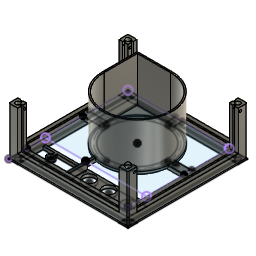
frame_top (Autodesk Fusion 360 design; units mm, degrees)
Autodesk Fusion 360 part; units mm, degrees
note: some values were not read from the file. Set by a fixed rule: which sketch regions a step uses.
sketch "Skizze1" plane through (0, 0, 0) normal (0, 0, 1) x (1, 0, 0)
  line L0 (0, 0) -> (160, 0)
  line L1 (160, 0) -> (160, 160)
  line L2 (160, 160) -> (0, 160)
  line L3 (0, 160) -> (0, 0)
  line L4 (0, 0) -> (12, 0)
  line L5 (12, 0) -> (12, 12)
  line L6 (12, 12) -> (0, 12)
  line L7 (0, 12) -> (0, 0)
  line L8 (160, 0) -> (148, 0)
  line L9 (148, 0) -> (148, 12)
  line L10 (148, 12) -> (160, 12)
  line L11 (160, 12) -> (160, 0)
  line L12 (160, 160) -> (148, 160)
  line L13 (148, 160) -> (148, 148)
  line L14 (148, 148) -> (160, 148)
  line L15 (160, 148) -> (160, 160)
  line L16 (0, 160) -> (12, 160)
  line L17 (12, 160) -> (12, 148)
  line L18 (12, 148) -> (0, 148)
  line L19 (0, 148) -> (0, 160)
  line L20 (12, 148) -> (148, 148)
  line L21 (148, 148) -> (148, 12)
  line L22 (148, 12) -> (12, 12)
  line L23 (12, 12) -> (12, 148)
  circle A0 centre (154, 154) radius 3
  circle A1 centre (6, 154) radius 3
  circle A2 centre (6, 6) radius 3
  circle A3 centre (154, 6) radius 3
  line L24 (4.9, 148) -> (7.1, 148)
  line L25 (7.1, 148) -> (7.1, 12)
  line L26 (7.1, 12) -> (4.9, 12)
  line L27 (4.9, 12) -> (4.9, 148)
  line L28 (152.9, 148) -> (155.1, 148)
  line L29 (155.1, 148) -> (155.1, 12)
  line L30 (155.1, 12) -> (152.9, 12)
  line L31 (152.9, 12) -> (152.9, 148)
  line L32 (12, 155.1) -> (148, 155.1)
  line L33 (148, 155.1) -> (148, 152.9)
  line L34 (148, 152.9) -> (12, 152.9)
  line L35 (12, 152.9) -> (12, 155.1)
  line L36 (12, 7.1) -> (148, 7.1)
  line L37 (148, 7.1) -> (148, 4.9)
  line L38 (148, 4.9) -> (12, 4.9)
  line L39 (12, 4.9) -> (12, 7.1)
  line L40 (148, 155.1) -> (150, 155.1)
  line L41 (150, 155.1) -> (150, 152.9)
  line L42 (150, 152.9) -> (148, 152.9)
  line L43 (148, 152.9) -> (148, 155.1)
  line L44 (152.9, 148) -> (155.1, 148)
  line L45 (155.1, 148) -> (155.1, 150)
  line L46 (155.1, 150) -> (152.9, 150)
  line L47 (152.9, 150) -> (152.9, 148)
  line L48 (12, 155.1) -> (10, 155.1)
  line L49 (10, 155.1) -> (10, 152.9)
  line L50 (10, 152.9) -> (12, 152.9)
  line L51 (12, 152.9) -> (12, 155.1)
  line L52 (4.9, 148) -> (7.1, 148)
  line L53 (7.1, 148) -> (7.1, 150)
  line L54 (7.1, 150) -> (4.9, 150)
  line L55 (4.9, 150) -> (4.9, 148)
  line L56 (12, 4.9) -> (10, 4.9)
  line L57 (10, 4.9) -> (10, 7.1)
  line L58 (10, 7.1) -> (12, 7.1)
  line L59 (12, 7.1) -> (12, 4.9)
  line L60 (4.9, 12) -> (7.1, 12)
  line L61 (7.1, 12) -> (7.1, 10)
  line L62 (7.1, 10) -> (4.9, 10)
  line L63 (4.9, 10) -> (4.9, 12)
  line L64 (148, 4.9) -> (150, 4.9)
  line L65 (150, 4.9) -> (150, 7.1)
  line L66 (150, 7.1) -> (148, 7.1)
  line L67 (148, 7.1) -> (148, 4.9)
  line L68 (152.9, 12) -> (155.1, 12)
  line L69 (155.1, 12) -> (155.1, 10)
  line L70 (155.1, 10) -> (152.9, 10)
  line L71 (152.9, 10) -> (152.9, 12)
  line L72 (148, 17) -> (66, 17)
  line L73 (66, 17) -> (66, 37)
  line L74 (66, 37) -> (148, 37)
  line L75 (148, 37) -> (148, 17)
  circle A4 centre (133, 27) radius 8.1
  circle A5 centre (107, 27) radius 8.1
  circle A6 centre (81, 27) radius 8.1
  line L76 (66, 37) -> (12, 37)
  line L77 (12, 37) -> (12, 34)
  line L78 (12, 34) -> (66, 34)
  line L79 (66, 34) -> (66, 37)
  line L80 (66, 17) -> (12, 17)
  line L81 (12, 17) -> (12, 20)
  line L82 (12, 20) -> (66, 20)
  line L83 (66, 20) -> (66, 17)
  circle A7 centre (29, 27) radius 3.6
  circle A8 centre (29, 27) radius 5
  line L84 (27.5, 34) -> (30.5, 34)
  line L85 (30.5, 34) -> (30.5, 12)
  line L86 (30.5, 12) -> (27.5, 12)
  line L87 (27.5, 12) -> (27.5, 34)
  dimension "d1" = 160
  dimension "d2" = 160
  dimension "d3" = 12
  dimension "d4" = 12
  dimension "d5" = 12
  dimension "d6" = 12
  dimension "d7" = 12
  dimension "d8" = 12
  dimension "d9" = 12
  dimension "d10" = 12
  dimension "d11" = 136
  dimension "d12" = 136
  dimension "d13" = 6
  dimension "d14" = 6
  dimension "d15" = 6
  dimension "d16" = 6
  dimension "d17" = 6
  dimension "d18" = 6
  dimension "d19" = 6
  dimension "d20" = 6
  dimension "d21" = 6
  dimension "d22" = 6
  dimension "d23" = 6
  dimension "d24" = 6
  dimension "d25" = 2.2
  dimension "d26" = 136
  dimension "d27" = 4.9
  dimension "d28" = 2.2
  dimension "d29" = 136
  dimension "d30" = 4.9
  dimension "d31" = 136
  dimension "d32" = 2.2
  dimension "d33" = 4.9
  dimension "d34" = 136
  dimension "d35" = 2.2
  dimension "d36" = 4.9
  dimension "d37" = 2
  dimension "d38" = 2.2
  dimension "d39" = 2.2
  dimension "d40" = 2
  dimension "d41" = 2
  dimension "d42" = 2.2
  dimension "d43" = 2.2
  dimension "d44" = 2
  dimension "d45" = 2
  dimension "d46" = 2.2
  dimension "d47" = 2.2
  dimension "d48" = 2
  dimension "d49" = 2
  dimension "d50" = 2.2
  dimension "d51" = 2.2
  dimension "d52" = 2
  dimension "d53" = 82
  dimension "d54" = 20
  dimension "d55" = 37
  dimension "d56" = 16.2
  dimension "d57" = 16.2
  dimension "d58" = 16.2
  dimension "d59" = 10
  dimension "d60" = 10
  dimension "d61" = 10
  dimension "d62" = 15
  dimension "d63" = 26
  dimension "d64" = 26
  dimension "d65" = 3
  dimension "d66" = 54
  dimension "d67" = 3
  dimension "d68" = 7.2
  dimension "d69" = 10
  dimension "d70" = 17
  dimension "d71" = 10
  dimension "d72" = 3
  dimension "d73" = 15.5
  constraint horizontal L0
  constraint vertical L1
  constraint horizontal L2
  constraint vertical L3
  constraint coincident L0.start L3.end
  constraint horizontal L4
  constraint vertical L5
  constraint horizontal L6
  constraint vertical L7
  constraint horizontal L8
  constraint vertical L9
  constraint horizontal L10
  constraint vertical L11
  constraint horizontal L12
  constraint vertical L13
  constraint horizontal L14
  constraint vertical L15
  constraint horizontal L16
  constraint vertical L17
  constraint horizontal L18
  constraint vertical L19
  constraint horizontal L20
  constraint vertical L21
  constraint horizontal L22
  constraint vertical L23
  constraint horizontal L24
  constraint vertical L25
  constraint horizontal L26
  constraint vertical L27
  constraint coincident L18 L24.start
  constraint horizontal L28
  constraint vertical L29
  constraint horizontal L30
  constraint vertical L31
  constraint coincident L14 L28.start
  constraint horizontal L32
  constraint vertical L33
  constraint horizontal L34
  constraint vertical L35
  constraint coincident L17 L32.start
  constraint horizontal L36
  constraint vertical L37
  constraint horizontal L38
  constraint vertical L39
  constraint coincident L5 L36.start
  constraint horizontal L40
  constraint vertical L41
  constraint horizontal L42
  constraint vertical L43
  constraint horizontal L44
  constraint vertical L45
  constraint horizontal L46
  constraint vertical L47
  constraint horizontal L48
  constraint vertical L49
  constraint horizontal L50
  constraint vertical L51
  constraint horizontal L52
  constraint vertical L53
  constraint horizontal L54
  constraint vertical L55
  constraint horizontal L56
  constraint vertical L57
  constraint horizontal L58
  constraint vertical L59
  constraint horizontal L60
  constraint vertical L61
  constraint horizontal L62
  constraint vertical L63
  constraint horizontal L64
  constraint vertical L65
  constraint horizontal L66
  constraint vertical L67
  constraint horizontal L68
  constraint vertical L69
  constraint horizontal L70
  constraint vertical L71
  constraint horizontal L72
  constraint vertical L73
  constraint horizontal L74
  constraint vertical L75
  constraint coincident L21 L72.start
  constraint horizontal L76
  constraint vertical L77
  constraint horizontal L78
  constraint vertical L79
  constraint horizontal L80
  constraint vertical L81
  constraint horizontal L82
  constraint vertical L83
  constraint concentric A7 A8
  constraint horizontal L84
  constraint vertical L85
  constraint horizontal L86
  constraint vertical L87
  constraint coincident L78 L84.start
  measures "d1" distance of L1 L3
  measures "d2" distance of L0 L2
  measures "d3" distance of L0.start L4.end
  measures "d4" distance of L0.start L6.end
  measures "d5" distance of L0.end L8.end
  measures "d6" distance of L0.end L10.end
  measures "d7" distance of L1.end L12.end
  measures "d8" distance of L1.end L14.end
  measures "d9" distance of L2.end L16.end
  measures "d10" distance of L2.end L18.end
  measures "d11" distance of L17.end L13.end
  measures "d12" distance of L17.end L5.end
  measures "d13" diameter of A0
  measures "d14" diameter of A1
  measures "d15" diameter of A2
  measures "d16" diameter of A3
  measures "d17" distance of L2 A0.centre
  measures "d18" distance of L15 A0.centre
  measures "d19" distance of L1 A3.centre
  measures "d20" distance of L8 A3.centre
  measures "d21" distance of L3 A2.centre
  measures "d22" distance of L4 A2.centre
  measures "d23" distance of L19 A1.centre
  measures "d24" distance of L2 A1.centre
  measures "d25" distance of L24.start L24.end
  measures "d26" distance of L24.start L26.end
  measures "d27" distance of L3 L27
  measures "d28" distance of L28.start L28.end
  measures "d29" distance of L28.start L30.end
  measures "d30" distance of L1 L29
  measures "d31" distance of L32.start L32.end
  measures "d32" distance of L32.start L34.end
  measures "d33" distance of L2 L32
  measures "d34" distance of L36.start L36.end
  measures "d35" distance of L36.start L38.end
  measures "d36" distance of L0 L38
  measures "d37" distance of L32.end L40.end
  measures "d38" distance of L32.end L33.end
  measures "d39" distance of L28.start L28.end
  measures "d40" distance of L28.start L46.end
  measures "d41" distance of L32.start L48.end
  measures "d42" distance of L32.start L34.end
  measures "d43" distance of L24.start L24.end
  measures "d44" distance of L24.start L54.end
  measures "d45" distance of L38.end L56.end
  measures "d46" distance of L38.end L36.start
  measures "d47" distance of L26.end L25.end
  measures "d48" distance of L26.end L62.end
  measures "d49" distance of L37.end L64.end
  measures "d50" distance of L37.end L36.end
  measures "d51" distance of L30.end L29.end
  measures "d52" distance of L30.end L70.end
  measures "d53" distance of L72.start L72.end
  measures "d54" distance of L72.start L74.end
  measures "d55" distance of L0 L74
  measures "d56" diameter of A4
  measures "d57" diameter of A5
  measures "d58" diameter of A6
  measures "d59" distance of L72 A4.centre
  measures "d60" distance of L72 A5.centre
  measures "d61" distance of L72 A6.centre
  measures "d62" distance of L21 A4.centre
  measures "d63" distance of A4.centre A5.centre
  measures "d64" distance of A5.centre A6.centre
  measures "d65" distance of L73.end L78.end
  measures "d66" distance of L72.end L80.end
  measures "d67" distance of L72.end L82.end
  measures "d68" diameter of A7
  measures "d69" diameter of A8
  measures "d70" distance of L23 A7.centre
  measures "d71" distance of L80 A7.centre
  measures "d72" distance of L84.start L84.end
  measures "d73" distance of L23 L87
ref_plane "Arbeitsebene1" through (80, 92.5, 12) normal (0, 0, 1) x (1, 0, 0)
sketch "Skizze2" plane through (80, 92.5, 12) normal (0, 0, 1) x (1, 0, 0)
  line L0 (-68, 55.5) -> (68, 55.5)
  line L1 (-14, -55.5) -> (68, -55.5)
  line L2 (-68, -80.5) -> (-68, 55.5)
  line L3 (68, 55.5) -> (68, -80.5)
  line L4 (-14, -55.5) -> (-68, -55.5)
  circle A0 centre (0, 0) radius 38.5
  circle A1 centre (0, 0) radius 44.5
  circle A2 centre (0, 0) radius 46.5
  circle A3 centre (0, 0) radius 41.5 construction
  circle A4 centre (41.5, 0) radius 2
  circle A5 centre (0, 41.5) radius 2
  circle A6 centre (-41.5, 0) radius 2
  circle A7 centre (0, -41.5) radius 2
  line L5 (0, 55.5) -> (0, 41.5) construction
  line L6 (0, 41.5) -> (5, 41.5) construction
  line L7 (5, 55.5) -> (5, 46.2304)
  line L8 (-5, 55.5) -> (-5, 46.2304)
  line L9 (41.5, 0) -> (51.5, 0) construction
  line L10 (41.5, 0) -> (41.5, -5) construction
  line L11 (68, -5) -> (46.2304, -5)
  line L12 (68, 5) -> (46.2304, 5)
  line L13 (-41.5, 0) -> (-51.5, 0) construction
  line L14 (-41.5, 0) -> (-41.5, -5) construction
  line L15 (-68, -5) -> (-46.2304, -5)
  line L16 (-68, 5) -> (-46.2304, 5)
  line L17 (-14, -55.5) -> (-14, -44.3424)
  line L18 (-14, -55.5) -> (-11, -55.5)
  line L19 (-11, -55.5) -> (-11, -45.1802)
  line L20 (-68, -80.5) -> (68, -80.5) construction
  line L21 (-14, -55.5) -> (-11, -55.5)
  line L22 (-11, -55.5) -> (-11, -80.5)
  line L23 (-11, -80.5) -> (-14, -80.5)
  line L24 (-14, -80.5) -> (-14, -55.5)
  line L25 (0, 46.5) -> (-46.5, 46.5)
  line L26 (-46.5, 0) -> (-46.5, 46.5)
  line L27 (-44.5, 0) -> (-44.5, 46.5)
  line L28 (0, 44.5) -> (-46.5, 44.5)
  line L29 (46.2304, 5) -> (44.2182, 5)
  line L30 (46.2304, -5) -> (44.2182, -5)
  line L31 (5, 46.2304) -> (5, 44.2182)
  line L32 (-5, 46.2304) -> (-5, 44.2182)
  line L33 (-46.2304, 5) -> (-44.2182, 5)
  line L34 (-46.2304, -5) -> (-44.2182, -5)
  line L35 (-14, -44.3424) -> (-14, -42.2404)
  line L36 (-11, -45.1802) -> (-11, -43.119)
  dimension "d75" = 77
  dimension "d76" = 89
  dimension "d77" = 93
  dimension "d78" = 83
  dimension "d79" = 4
  dimension "d81" = 360
  dimension "d82" = 26.5
  dimension "d83" = 5
  dimension "d84" = 10
  dimension "d85" = 5
  dimension "d86" = 10
  dimension "d87" = 5
  dimension "d88" = 3
  dimension "d89" = 3
  dimension "d90" = 25
  dimension "d91" = 5
  dimension "d92" = 5
  dimension "d93" = 5
  constraint coincident A0.centre A1.centre
  constraint concentric A0 A2
  constraint coincident A3 A4.centre
  constraint midpoint L0 L5.start
  constraint coincident A5.centre L5.end
  constraint perpendicular L5 L6
  constraint coincident L0 L7.start
  constraint coincident A2 L7.end
  constraint perpendicular L0 L7
  constraint symmetric L5 L7.start L8.start
  constraint symmetric L5 L7.end L8.end
  constraint coincident A4.centre L9.start
  constraint horizontal L9
  constraint tangent A3 L10
  constraint perpendicular L9 L10
  constraint coincident L3 L11.start
  constraint coincident A2 L11.end
  constraint perpendicular L3 L11
  constraint symmetric L9 L11.start L12.start
  constraint symmetric L9 L11.end L12.end
  constraint coincident A6.centre L13.start
  constraint horizontal L13
  constraint perpendicular L13 L14
  constraint coincident L2 L15.start
  constraint coincident A2 L15.end
  constraint perpendicular L2 L15
  constraint symmetric L13 L15.start L16.start
  constraint symmetric L13 L15.end L16.end
  constraint coincident L1.start L4.start
  constraint coincident A2 L17.end
  constraint perpendicular L1 L17
  constraint perpendicular L17 L18
  constraint coincident A2 L19.end
  constraint perpendicular L1 L19
  constraint coincident L2.start L20.start
  constraint coincident L3.end L20.end
  constraint horizontal L21
  constraint vertical L22
  constraint horizontal L23
  constraint vertical L24
  constraint coincident A2 L25.start
  constraint coincident L5 L25.start
  constraint tangent A2 L25
  constraint midpoint L13 L26.start
  constraint tangent A2 L26
  constraint perpendicular L25 L26
  constraint coincident L13 L27.start
  constraint coincident A1 L27.start
  constraint tangent A1 L27
  constraint coincident A1 L28.start
  constraint coincident L5 L28.start
  constraint tangent A1 L28
  constraint coincident L26 L28.end
  constraint coincident L25 L27.end
  constraint coincident A1 L29.end
  constraint parallel L12 L29
  constraint coincident A1 L30.end
  constraint parallel L11 L30
  constraint coincident A1 L31.end
  constraint parallel L7 L31
  constraint coincident A1 L32.end
  constraint perpendicular L28 L32
  constraint coincident A1 L33.end
  constraint perpendicular L27 L33
  constraint coincident A1 L34.end
  constraint parallel L15 L34
  constraint coincident A1 L35.end
  constraint parallel L17 L35
  constraint parallel L19 L36
  constraint coincident A1 L36.end
  measures "d75" diameter of A0
  measures "d76" diameter of A1
  measures "d77" diameter of A2
  measures "d78" diameter of A3
  measures "d79" diameter of A4
  measures "d82" distance of L3 A4.centre
  measures "d83" distance of A5.centre L6.end
  measures "d84" distance of A4.centre L9.end
  measures "d85" distance of A4.centre L10.end
  measures "d86" distance of A6.centre L13.end
  measures "d87" distance of A6.centre L14.end
  measures "d88" distance of L1.start L18.end
  measures "d89" distance of L1.start L18.end
  measures "d90" distance of L1.start L23.end
  measures "d91" distance of A0.centre L7
  measures "d92" distance of A0.centre L11
  measures "d93" distance of A0.centre L15
extrude "Extrusion1" add sketch "Skizze2" against normal blind 4.9 contours L0 A2 L7 L8 L25 | L2 A2 L15 L16 L26 | A2 L8 L25 | A2 L16 L26 | A1 A2 L28 L31 L32 | A1 A2 L27 L33 L34 | L3 A2 L11 L12 | A1 A2 L29 L30 | A1 | A1 L28 L32 | L1 A2 L17 L18 L19 L21 | A1 A2 L35 L36 | A1 L27 L33 makes body 1
extrude "Extrusion2" add sketch "Skizze1" along normal blind 65 separate body contours L0 L3 L4 L5 L6 L7 L56 L57 L58 L61 L62 L63 | L0 L1 L8 L9 L10 L11 L64 L65 L66 L69 L70 L71 | L2 L3 L16 L17 L18 L19 L48 L49 L50 L53 L54 L55 | L1 L2 L12 L13 L14 L15 L40 L41 L42 L45 L46 L47 makes body 2 at (156.8191, 155.0261, 43.3333) makes body 3 at (153.0445, 3.1562, 21.6667) makes body 4 at (3.1809, 155.0261, 43.3333) makes body 5 at (8.9851, 5.7013, 21.6667)
extrude "Extrusion3" add sketch "Skizze1" along normal blind 12 separate body contours L0 L5 L9 L38 | L3 L6 L18 L27 | L1 L10 L14 L29 | L2 L13 L17 L32 makes body 6 at (0, 102.6667, 8) makes body 7 at (155.1, 102.6667, 8) makes body 8 at (102.6667, 160, 8) makes body 9 at (102.6667, 4.9, 8)
extrude "Extrusion4" add sketch "Skizze1" along normal blind 12 separate body contours L5 L9 L22 L36 L86 | L6 L18 L23 L25 L77 L81 | L10 L14 L21 L31 L75 | L13 L17 L20 L34 makes body 10 at (102.6667, 152.9, 8)
extrude "Extrusion5" add sketch "Skizze1" along normal blind 10 separate body contours L5 L39 L56 L57 L58 L59 | L5 L9 L36 L37 L38 L39 L59 L67 | L6 L18 L24 L25 L26 L27 L52 L60 | L6 L26 L60 L61 L62 L63 | L9 L37 L64 L65 L66 L67 | L18 L24 L52 L53 L54 L55 | L10 L30 L68 L69 L70 L71 | L10 L14 L28 L29 L30 L31 L44 L68 | L13 L17 L32 L33 L34 L35 L43 L51 | L17 L35 L48 L49 L50 L51 | L14 L28 L44 L45 L46 L47 | L13 L33 L40 L41 L42 L43 makes body 11 at (155.1, 103.3333, 3.3333) makes body 12 at (4.9, 103.3333, 3.3333) makes body 13 at (56.6667, 152.9, 3.3333) makes body 14 at (103.3333, 7.1, 3.3333)
extrude "Extrusion6" add sketch "Skizze2" against normal blind 3 separate body contours A2 L8 L25 L27 L28 | A2 L16 L26 L27 L28 | A1 A2 L29 L31 | A2 L28 L32 | L25 L26 L27 L28 | A1 A2 L34 L35 | A2 L27 L33 | A1 A2 L27 L28 L32 L33 | A2 L27 L28 | A1 A2 L30 L36 makes body 15 at (92.904, 47.8263, 10) makes body 16 at (47.034, 59.7053, 10) makes body 17 at (89.1511, 138.0907, 10) makes body 18 at (43.5811, 128.9189, 12)
extrude "Extrusion7" add sketch "Skizze2" along normal blind 60 separate body contours A2 L8 L25 | A2 L8 L25 L27 L28 | A2 L16 L26 L27 L28 | A2 L16 L26 | A1 A2 L28 L31 L32 | A1 A2 L29 L31 | A2 L28 L32 | L25 L26 L27 L28 | A1 A2 L34 L35 | A1 A2 L27 L33 L34 | A2 L27 L33 | A1 A2 L29 L30 | A1 A2 L35 L36 | A1 A2 L30 L36 makes body 19
extrude "Extrusion8" add sketch "Skizze1" along normal blind 4 separate body contours L22 L80 L85 L86 L87 | L23 L80 L81 L82 L87 | L21 L72 L73 L74 L75 L79 L83 | L80 L82 L85 L87 | L23 L73 L76 L77 L78 L79 L84 | L73 L80 L82 L83 L85 | L82 A8 L85 L87 | A7 A8 L85 L87 | A7 A8 L87 | L78 A8 L84 L85 L87 | A7 A8 L85 | A7 A8 L85 L87 makes body 20
extrude "Extrusion9" add sketch "Skizze1" along normal blind 55 separate body contours A0 | A1 | A2 | A3 makes body 21 at (153.0445, 3.1562, 18.3333) makes body 22 at (3.1809, 155.0261, 36.6667) makes body 23 at (8.9851, 5.7013, 18.3333) makes body 24 at (156.7644, 155.1653, 36.6667)
extrude "Extrusion10" add sketch "Skizze2" against normal blind 8 separate body contours L1 L18 L21 L22 L23 L24 makes body 25
sketch "Skizze3" plane through (0, 0, 0) normal (-1, 0, 0) x (0, -1, 0)
  line L0 (-12, 0) -> (0, 0)
  line L1 (0, 0) -> (0, 65)
  line L2 (0, 65) -> (-12, 65)
  line L3 (-12, 65) -> (-12, 0)
  line L4 (-12, 65) -> (-9, 65) construction
  line L5 (-9, 65) -> (-9, 60) construction
  circle A0 centre (-9, 60) radius 1.5
  dimension "d114" = 3
  dimension "d115" = 5
  dimension "d116" = 3
  constraint coincident L2.end L3.start
  constraint perpendicular L3 L4
  constraint perpendicular L4 L5
  constraint coincident L5.end A0.centre
  measures "d114" distance of L2.end L4.end
  measures "d115" distance of L4.end L5.end
  measures "d116" diameter of A0
extrude "Extrusion11" cut sketch "Skizze3" against normal through all contours A0 bodies 3 5
sketch "Skizze4" plane through (0, 0, 0) normal (1, 0, 0) x (0, 1, 0)
  line L0 (148, 65) -> (151, 65) construction
  line L1 (151, 65) -> (151, 60) construction
  circle A0 centre (151, 60) radius 1.5
  dimension "d118" = 3
  dimension "d119" = 5
  dimension "d120" = 3
  constraint horizontal L0
  constraint perpendicular L0 L1
  constraint coincident L1.end A0.centre
  measures "d118" distance of L0.start L0.end
  measures "d119" distance of L0.end L1.end
  measures "d120" diameter of A0
extrude "Extrusion12" cut sketch "Skizze4" along normal through all bodies 2 4
combine "Kombinieren1" operation add target body 1 tool bodies 10 11 12 18 19 21 14 20 15 16 13 17 3 2 5 6 7 8 9 4 23 24 25 22
move_face "Flächen versetzen1" offset -0.1 8 faces at (3.2074, 152.904, 60) (6.0272, 150.7768, 61.4833) (3.2074, 7.096, 60) (6.0272, 9.2232, 61.4833) (151.2074, 7.096, 60) (154.0272, 9.2232, 61.4833) (156.7926, 152.904, 60) (154.0272, 150.7768, 61.4833) on bodies 1
fillet "Abrundung1" radius 1.5 8 edges at (160, 0, 32.5) (80, 0, 0) (160, 80, 0) (160, 160, 32.5) (80, 160, 0) (0, 160, 32.5) (0, 80, 0) (0, 0, 32.5) on bodies 1
fillet "Abrundung2" radius 1.5 1 edges at (33.5, 139, 40.5) on bodies 1
